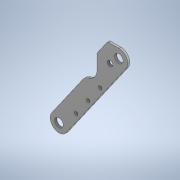
# Autodesk Inventor part: BackLink_frame
Saved by Autodesk Inventor 2020 (Build 240168000, 168)
## iProperties
Created: 2021-10-03
Part Number: BackLink_frame
Material: GFRP
Document SubType Name: Modeling
Designer: Masato Kubotera
Density: 1.75 g/cm^3
Appearance: 滑らか - 標準の灰色
Description: GFRP T2
Mass: 6.44398 g
Surface Area: 43.7409 cm^2
Volume: 3.68228 cm^3
Author: Masato Kubotera
Autodesk Inventor part; units mm, degrees
ref_plane "YZ Plane" through (0, 0, 0) normal (1, 0, 0) x (0, 1, 0)
ref_plane "XZ Plane" through (0, 0, 0) normal (0, 1, 0) x (-1, 0, 0)
ref_plane "XY Plane" through (0, 0, 0) normal (0, 0, 1) x (1, 0, 0)
derived "Link_basis.ipt"
sketch "スケッチ1" plane through (0, 0, 0) normal (0, 0, 1) x (1, 0, 0)
  circle A0 centre (0, 0) radius 6
  circle A1 centre (-57.3576, -81.9152) radius 4
  arc A2 (-64.3515, -81.6228) -> (-57.3576, -88.9152) centre (-57.3576, -81.9152) ccw
  arc A3 (2.9295, -10.6027) -> (-4.5598, 10.0104) centre (0, 0) ccw
  line L0 (-61.4483, -42.4277) -> (-35.6374, -5.5658) construction
  line L1 (-35.6374, -5.5658) -> (-31.5416, -8.4337) construction
  line L2 (-31.5416, -8.4337) -> (-57.3525, -45.2955) construction
  line L3 (-57.3525, -45.2955) -> (-61.4483, -42.4277) construction
  line L4 (-61.4483, -42.4277) -> (-31.5416, -8.4337) construction
  line L5 (-35.6374, -5.5658) -> (-57.3525, -45.2955) construction
  line L6 (-59.4004, -43.8616) -> (-33.5895, -6.9998) construction
  circle A4 centre (-56.5325, -39.7658) radius 1.6
  circle A5 centre (-46.495, -25.4307) radius 1.6
  line L7 (-48.5428, -23.9967) -> (-44.4471, -26.8646) construction
  circle A6 centre (-36.4574, -11.0955) radius 1.6
  line L8 (-62.677, -41.5673) -> (-36.8661, -4.7054)
  line L9 (-36.8661, -4.7054) -> (-4.5598, 10.0104)
  line L10 (-62.677, -41.5673) -> (-64.3515, -81.6228)
  line L11 (-32.3614, -57.0111) -> (-2.5989, -14.5058)
  line L12 (0, 0) -> (32, 0) construction
  line L13 (32, 0) -> (32, 20) construction
  circle A7 centre (32, 20) radius 4
  arc A8 (38.9218, 15.1533) -> (32, 28.45) centre (32, 20) ccw
  line L14 (32, 20) -> (32, 37) construction
  circle A9 centre (32, 37) radius 4 construction
  circle A10 centre (32, 37) radius 8.45 construction
  line L15 (-57.3576, -81.9152) -> (0, 0) construction
  circle A11 centre (0, 0) radius 8.5 construction
  circle A12 centre (6.0104, 6.0104) radius 1.4
  circle A13 centre (32, 20) radius 7 construction
  arc A14 (-64.3515, -81.6228) -> (-53.3426, -76.1811) centre (-57.3576, -81.9152) ccw construction
  line L16 (-51.6236, -85.9302) -> (-33.7808, -60.4482)
  line L17 (38.9218, 15.1533) -> (-18.4358, -66.7619)
  line L18 (32, 20) -> (-25.3576, -61.9152) construction
  circle A15 centre (-25.3576, -61.9152) radius 4
  circle A16 centre (-25.3576, -61.9152) radius 8 construction
  arc A17 (2.9744, -10.6941) -> (11.1, 0) centre (0, 0) ccw
  line L19 (25.0782, 24.8467) -> (10.3989, 3.8825) construction
  line L20 (-2.5375, -14.5926) -> (-32.2795, -57.0685)
  arc A18 (-32.2795, -57.0685) -> (-18.4358, -66.7619) centre (-25.3576, -61.9152) ccw
  arc A19 (-32.3614, -57.0111) -> (-32.5799, -66.4914) centre (-25.3576, -61.9152) ccw
  line L21 (-6.0104, 6.0104) -> (0, 0) construction
  circle A20 centre (-6.0104, 6.0104) radius 1.4
  circle A21 centre (-6.0104, -6.0104) radius 1.4
  circle A22 centre (6.0104, -6.0104) radius 1.4
  line L22 (-12.2888, -46.6506) -> (2.0506, -26.1718) construction
  line L23 (2.0506, -26.1718) -> (6.1464, -29.0397) construction
  line L24 (6.1464, -29.0397) -> (-8.193, -49.5185) construction
  line L25 (-8.193, -49.5185) -> (-12.2888, -46.6506) construction
  line L26 (-12.2888, -46.6506) -> (6.1464, -29.0397) construction
  line L27 (2.0506, -26.1718) -> (-8.193, -49.5185) construction
  line L28 (4.0985, -27.6058) -> (-10.2409, -48.0846) construction
  line L29 (-5.1191, -36.4112) -> (-1.0233, -39.2791) construction
  circle A23 centre (2.6646, -29.6537) radius 1.6
  circle A24 centre (-8.8069, -46.0367) radius 1.6
  line L30 (7.185, 8.4608) -> (11.1, 14.052)
  line L31 (32, 28.45) -> (21.1816, 28.45)
  arc A25 (32, 28.45) -> (25.0782, 24.8467) centre (32, 20) ccw construction
  line L32 (-32.5799, -66.4914) -> (-48.2812, -88.9152)
  line L33 (-57.3576, -88.9152) -> (-48.2812, -88.9152)
  arc A26 (-57.3576, -88.9152) -> (-51.6236, -85.9302) centre (-57.3576, -81.9152) ccw construction
  line L34 (20.5285, 3.617) -> (-5.6844, 21.9714) construction
  line L35 (-5.6844, 21.9714) -> (14.1146, 2.1724) construction
  line L36 (14.1146, 2.1724) -> (23.6605, 11.7184) construction
  line L37 (14.1146, 2.1724) -> (4.5687, -7.3735)
  arc A27 (5.2542, -9.7777) -> (6.4162, -9.0577) centre (4.5687, -7.3735) ccw
  line L38 (11.1, 0) -> (11.1, 14.052)
  line L39 (11.1, 14.052) -> (21.1816, 28.45)
  arc A28 (11.1, 0) -> (7.185, 8.4608) centre (0, 0) ccw construction
  line L40 (0, 0) -> (6.0104, 6.0104)
  circle A29 centre (23.6605, 11.7184) radius 2.5
  line L41 (0.6167, -28.2197) -> (4.7125, -31.0876) construction
  line L42 (13.5222, -9.7888) -> (-0.8172, -30.2676) construction
  line L43 (3.2785, -33.1355) -> (17.6179, -12.6567) construction
  line L44 (6.3525, -20.0282) -> (10.4482, -22.8961) construction
  line L45 (17.6179, -12.6567) -> (13.5222, -9.7888) construction
  circle A30 centre (14.1361, -13.2706) radius 1.6
  line L46 (-0.8172, -30.2676) -> (3.2785, -33.1355) construction
  arc A31 (2.9295, -10.6027) -> (-2.5989, -14.5058) centre (5.5927, -20.2416) ccw
  arc A32 (2.9744, -10.6941) -> (-2.5375, -14.5926) centre (5.654, -20.3284) ccw
  point P0 (-0.1434, -10.9991)
  point P1 (-0.0917, -11.0996)
  point P2 (-3.0712, -37.8452)
  dimension "d15" = 32
  dimension "d16" = 20
  dimension "d17" = 20
  dimension "d18" = 32
  dimension "d22" = 28
  dimension "d23" = 10
  dimension "d24" = 13.5
  dimension "d25" = 13.5
  dimension "d27" = 2.5
  dimension "d28" = 5
  measures "d15" distance of L34.start L34.end
  measures "d16" distance of L34.start L13.end
  measures "d17" distance of L12.end L13.end
  measures "d18" distance of L12.start L12.end
  measures "d22" distance of L34.end L35.end
  measures "d23" angle of L35 L34
  measures "d24" distance of L35.end L36.end
  measures "d25" distance of L35.end L37.end
  measures "d27" radius of A27
  measures "d28" diameter of A29
extrude "押し出し1" add sketch "スケッチ1" along normal blind 2 contours L17 A18 L20 A32 A17 A27 L38 L39 L31 A8 | A17 A27
fillet "フィレット1" radius 2 2 edges at (21.1816, 28.45, 1) (11.1, 14.052, 1)
equation "\"d15\" = d18"
equation "\"d16\" = d17"
equation "\"d25\" = d24"
